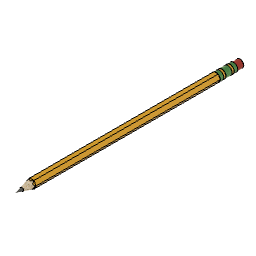
modeled_pencil (Autodesk Fusion 360 design; units mm, degrees)
Autodesk Fusion 360 part; units mm, degrees
sketch "Sketch1" plane through (0, 0, 0) normal (0, 1, 0) x (1, 0, 0)
  line L0 (1.8575, -3.2173) -> (3.715, 0)
  line L1 (3.715, 0) -> (1.8575, 3.2173)
  line L2 (1.8575, 3.2173) -> (-1.8575, 3.2173)
  line L3 (-1.8575, 3.2173) -> (-3.715, 0)
  line L4 (-3.715, 0) -> (-1.8575, -3.2173)
  line L5 (-1.8575, -3.2173) -> (1.8575, -3.2173)
  circle A0 centre (0, 0) radius 3.715
  dimension "d1" = 3.715
  constraint coincident A0.centre origin
  constraint horizontal L2
  constraint coincident L0.end A0
  measures "d1" distance of L0.start A0.centre
extrude "Extrude1" add sketch "Sketch1" along normal blind 160 makes body 1
sketch "Sketch3" plane through (0, 0, 0) normal (0, 0, 1) x (1, 0, 0)
  line L0 (0, 0) -> (0, -14.2)
  line L1 (0, -14.2) -> (3.715, 0)
  line L2 (3.715, 0) -> (0, 0)
  dimension "d4" = 14.2
  dimension "d10" = 3.715
  constraint coincident L0.start L2.end
  constraint vertical L0
  constraint perpendicular L0 L2
  measures "d4" distance of L0.start L0.end
  measures "d10" distance of L1.end L0.start
revolve "Revolve1" add sketch "Sketch3" angle 360 about axis through (0, 0, 0) along (0, -1, 0) separate body makes body 2
extrude "Extrude2" cut sketch "Sketch1" against normal blind 14 contours L5 A0 | L0 A0 | L1 A0 | L4 A0 | L2 A0 | L3 A0 bodies 2
extrude "Extrude3" cut sketch "Sketch1" along normal blind 160 contours L5 A0 | L0 A0 | L1 A0 | L4 A0 | L2 A0 | L3 A0 bodies 1
ref_plane "WorkPlane1" through (0, -8.75, 0) normal (0, 1, 0) x (1, 0, 0)
split "Split1" by plane through (0, -8.75, 0) normal (0, 1, 0) bodies 2 makes body 3 at (3.0891, -2.3333, 0.3091)
sketch "Sketch4" plane through (0, 160, 0) normal (0, 1, 0) x (-1, 0, 0)
  line L0 (-3.715, 0) -> (-1.8575, -3.2173)
  line L1 (-1.8575, -3.2173) -> (1.8575, -3.2173)
  line L2 (1.8575, -3.2173) -> (3.715, 0)
  line L3 (3.715, 0) -> (1.8575, 3.2173)
  line L4 (1.8575, 3.2173) -> (-1.8575, 3.2173)
  line L5 (-1.8575, 3.2173) -> (-3.715, 0)
  circle A0 centre (0, 0) radius 3.705
  dimension "d12" = 7.41
  constraint coincident A0.centre origin
  measures "d12" diameter of A0
extrude "Extrude4" add sketch "Sketch4" along normal blind 3.06 contours L0 L1 L2 L3 L4 L5 A0 | L0 A0 | L5 A0 | L1 A0 | L4 A0 | L2 A0 | L3 A0 bodies 1
sketch "Sketch5" plane through (0, 163.06, 0) normal (0, 1, 0) x (-1, 0, 0)
  circle A0 centre (0, 0) radius 3.705
  circle A1 centre (0, 0) radius 3.59
  dimension "d15" = 7.18
  constraint coincident A0.centre A1.centre
  measures "d15" diameter of A1
extrude "Extrude5" add sketch "Sketch5" along normal blind 1.78 contours A1 bodies 1
fillet "Fillet1" radius 0.1 1 edges at (3.4543, 163.06, -1.3398) on bodies 1
sketch "Sketch6" plane through (0, 164.84, 0) normal (0, 1, 0) x (-1, 0, 0)
  circle A0 centre (0, 0) radius 3.59
  circle A1 centre (0, 0) radius 3.705
  dimension "d20" = 7.41
  constraint coincident A0.centre A1.centre
  measures "d20" diameter of A1
extrude "Extrude6" add sketch "Sketch6" along normal blind 5.43 contours A0 | A1 bodies 1
fillet "Fillet2" radius 0.1 1 edges at (3.4543, 164.84, -1.3398) on bodies 1
sketch "Sketch7" plane through (0, 170.27, 0) normal (0, 1, 0) x (-1, 0, 0)
  circle A0 centre (0, 0) radius 3.705
  circle A1 centre (0, 0) radius 3.59
  dimension "d25" = 7.18
  constraint coincident A0.centre A1.centre
  measures "d25" diameter of A1
extrude "Extrude7" add sketch "Sketch7" along normal blind 1.78 contours A1 bodies 1
fillet "Fillet3" radius 0.1 1 edges at (3.4543, 170.27, -1.3398) on bodies 1
sketch "Sketch8" plane through (0, 172.05, 0) normal (0, 1, 0) x (-1, 0, 0)
  circle A0 centre (0, 0) radius 3.59
  circle A1 centre (0, 0) radius 3.705
  dimension "d30" = 7.41
  constraint coincident A0.centre A1.centre
  measures "d30" diameter of A1
extrude "Extrude8" add sketch "Sketch8" along normal blind 3.06 contours A0 | A1 bodies 1
fillet "Fillet4" radius 0.1 1 edges at (3.4543, 172.05, -1.3398) on bodies 1
sketch "Sketch9" plane through (0, 175.11, 0) normal (0, 1, 0) x (-1, 0, 0)
  circle A0 centre (0, 0) radius 3.705
  circle A1 centre (0, 0) radius 3.33
  dimension "d35" = 6.66
  constraint coincident A0.centre A1.centre
  measures "d35" diameter of A1
extrude "Extrude9" add sketch "Sketch9" along normal blind 6 contours A1 bodies 1
fillet "Fillet5" radius 0.5 1 edges at (3.1047, 181.11, -1.2042) on bodies 1
